Autodesk Fusion 360 part; units mm, degrees
(part 2 of 2)
  arc A538 (8.0741, 18.3325) -> (8.0737, 18.1922) centre (8.8652, 18.2601) ccw
  arc A539 (8.1154, 18.5393) -> (8.0741, 18.3325) centre (9.07, 18.2414) ccw
  arc A540 (8.1154, 18.5393) -> (8.0313, 18.7219) centre (7.9722, 18.584) ccw
  arc A541 (8.0313, 18.7219) -> (7.5594, 18.9174) centre (0, 0) ccw
  arc A542 (7.5594, 18.9174) -> (7.3708, 18.8477) centre (7.5037, 18.7781) ccw
  arc A543 (7.2538, 18.6723) -> (7.3708, 18.8477) centre (6.4851, 19.312) ccw
  arc A544 (7.1548, 18.5728) -> (7.2538, 18.6723) centre (6.6432, 19.1805) ccw
  arc A545 (6.6104, 18.4748) -> (7.1548, 18.5728) centre (6.7974, 18.9974) ccw
  arc A546 (6.2517, 18.896) -> (6.6104, 18.4748) centre (6.7974, 18.9974) ccw
  arc A547 (6.2384, 19.0357) -> (6.2517, 18.896) centre (7.0327, 19.0411) ccw
  arc A548 (6.2592, 19.2455) -> (6.2384, 19.0357) centre (7.2383, 19.0425) ccw
  arc A549 (6.2592, 19.2455) -> (6.1576, 19.419) centre (6.1123, 19.276) ccw
  arc A550 (6.1576, 19.419) -> (5.6687, 19.5672) centre (0, 0) ccw
  arc A551 (5.6687, 19.5672) -> (5.4879, 19.4795) centre (5.627, 19.4232) ccw
  arc A552 (5.3886, 19.2934) -> (5.4879, 19.4795) centre (4.561, 19.8547) ccw
  arc A553 (5.2999, 19.1847) -> (5.3886, 19.2934) centre (4.7312, 19.7393) ccw
  arc A554 (4.7677, 19.0338) -> (5.2999, 19.1847) centre (4.9026, 19.5722) ccw
  arc A555 (4.3695, 19.4177) -> (4.7677, 19.0338) centre (4.9026, 19.5722) ccw
  arc A556 (4.3425, 19.5555) -> (4.3695, 19.4177) centre (5.1325, 19.6388) ccw
  arc A557 (4.3426, 19.7663) -> (4.3425, 19.5555) centre (5.337, 19.6603) ccw
  arc A558 (4.3426, 19.7663) -> (4.2245, 19.929) centre (4.1935, 19.7822) ccw
  arc A559 (4.2245, 19.929) -> (3.7235, 20.0287) centre (0, 0) ccw
  arc A560 (3.7235, 20.0287) -> (3.5522, 19.9236) centre (3.6961, 19.8812) ccw
  arc A561 (3.4716, 19.7287) -> (3.5522, 19.9236) centre (2.5929, 20.2061) ccw
  arc A562 (3.394, 19.6118) -> (3.4716, 19.7287) centre (2.7736, 20.108) ccw
  arc A563 (2.8791, 19.4095) -> (3.394, 19.6118) centre (2.9606, 19.9584) ccw
  arc A564 (2.4452, 19.7525) -> (2.8791, 19.4095) centre (2.9606, 19.9584) ccw
  arc A565 (2.4048, 19.887) -> (2.4452, 19.7525) centre (3.1828, 20.0473) ccw
  arc A566 (2.3843, 20.0968) -> (2.4048, 19.887) centre (3.3842, 20.0888) ccw
  arc A567 (2.3843, 20.0968) -> (2.2508, 20.2471) centre (2.2343, 20.098) ccw
  arc A568 (2.2508, 20.2471) -> (1.7424, 20.2972) centre (0, 0) ccw
  arc A569 (1.7424, 20.2972) -> (1.5822, 20.1758) centre (1.7296, 20.1477) ccw
  arc A570 (1.5211, 19.974) -> (1.5822, 20.1758) centre (0.5999, 20.363) ccw
  arc A571 (1.4553, 19.85) -> (1.5211, 19.974) centre (0.7893, 20.283) ccw
  arc A572 (0.9628, 19.5982) -> (1.4553, 19.85) centre (0.99, 20.1525) ccw
  arc A573 (0.4973, 19.8971) -> (0.9628, 19.5982) centre (0.99, 20.1525) ccw
  arc A574 (0.444, 20.0269) -> (0.4973, 19.8971) centre (1.2025, 20.2627) ccw
  arc A575 (0.403, 20.2337) -> (0.444, 20.0269) centre (1.3989, 20.3237) ccw
  circle A576 centre (0, 0) radius 21.5
  dimension "d56" = 43
  constraint concentric A1 A576
  measures "d56" diameter of A576
extrude "Extruir10" add sketch "Boceto8" along normal blind 2 contours A0 A1 A2 A3 A4 A5 A6 A7 A8 A9 A10 A11 A12 A13 A14 A15 A16 A17 A18 A19 A20 A21 A22 A23 A24 A25 A26 A27 A28 A29 A30 A31 A32 A33 A34 A35 A36 A37 A38 A39 A40 A41 A42 A43 A44 A45 A46 A47 A48 A49 A50 A51 A52 A53 A54 A55 A56 A57 A58 A59 A60 A61 A62 A63 A64 A65 A66 A67 A68 A69 A70 A71 A72 A73 A74 A75 A76 A77 A78 A79 A80 A81 A82 A83 A84 A85 A86 A87 A88 A89 A90 A91 A92 A93 A94 A95 A96 A97 A98 A99 A100 A101 A102 A103 A104 A105 A106 A107 A108 A109 A110 A111 A112 A113 A114 A115 A116 A117 A118 A119 A120 A121 A122 A123 A124 A125 A126 A127 A128 A129 A130 A131 A132 A133 A134 A135 A136 A137 A138 A139 A140 A141 A142 A143 A144 A145 A146 A147 A148 A149 A150 A151 A152 A153 A154 A155 A156 A157 A158 A159 A160 A161 A162 A163 A164 A165 A166 A167 A168 A169 A170 A171 A172 A173 A174 A175 A176 A177 A178 A179 A180 A181 A182 A183 A184 A185 A186 A187 A188 A189 A190 A191 A192 A193 A194 A195 A196 A197 A198 A199 A200 A201 A202 A203 A204 A205 A206 A207 A208 A209 A210 A211 A212 A213 A214 A215 A216 A217 A218 A219 A220 A221 A222 A223 A224 A225 A226 A227 A228 A229 A230 A231 A232 A233 A234 A235 A236 A237 A238 A239 A240 A241 A242 A243 A244 A245 A246 A247 A248 A249 A250 A251 A252 A253 A254 A255 A256 A257 A258 A259 A260 A261 A262 A263 A264 A265 A266 A267 A268 A269 A270 A271 A272 A273 A274 A275 A276 A277 A278 A279 A280 A281 A282 A283 A284 A285 A286 A287 A288 A289 A290 A291 A292 A293 A294 A295 A296 A297 A298 A299 A300 A301 A302 A303 A304 A305 A306 A307 A308 A309 A310 A311 A312 A313 A314 A315 A316 A317 A318 A319 A320 A321 A322 A323 A324 A325 A326 A327 A328 A329 A330 A331 A332 A333 A334 A335 A336 A337 A338 A339 A340 A341 A342 A343 A344 A345 A346 A347 A348 A349 A350 A351 A352 A353 A354 A355 A356 A357 A358 A359 A360 A361 A362 A363 A364 A365 A366 A367 A368 A369 A370 A371 A372 A373 A374 A375 A376 A377 A378 A379 A380 A381 A382 A383 A384 A385 A386 A387 A388 A389 A390 A391 A392 A393 A394 A395 A396 A397 A398 A399 A400 A401 A402 A403 A404 A405 A406 A407 A408 A409 A410 A411 A412 A413 A414 A415 A416 A417 A418 A419 A420 A421 A422 A423 A424 A425 A426 A427 A428 A429 A430 A431 A432 A433 A434 A435 A436 A437 A438 A439 A440 A441 A442 A443 A444 A445 A446 A447 A448 A449 A450 A451 A452 A453 A454 A455 A456 A457 A458 A459 A460 A461 A462 A463 A464 A465 A466 A467 A468 A469 A470 A471 A472 A473 A474 A475 A476 A477 A478 A479 A480 A481 A482 A483 A484 A485 A486 A487 A488 A489 A490 A491 A492 A493 A494 A495 A496 A497 A498 A499 A500 A501 A502 A503 A504 A505 A506 A507 A508 A509 A510 A511 A512 A513 A514 A515 A516 A517 A518 A519 A520 A521 A522 A523 A524 A525 A526 A527 A528 A529 A530 A531 A532 A533 A534 A535 A536 A537 A538 A539 A540 A541 A542 A543 A544 A545 A546 A547 A548 A549 A550 A551 A552 A553 A554 A555 A556 A557 A558 A559 A560 A561 A562 A563 A564 A565 A566 A567 A568 A569 A570 A571 A572 A573 A574 A575 | A576 bodies 1
sketch "Boceto9" plane through (0, 0, 0) normal (0, 0, 1) x (1, 0, 0)
  circle A0 centre (0, 0) radius 21.5
  dimension "d59" = 43
  constraint coincident A0.centre origin
  measures "d59" diameter of A0
extrude "Extruir11" add sketch "Boceto9" against normal blind 7 bodies 1
move_body "Desplazar1" bodies 1 to x (1, 0, 0) y (0, 1, 0) z (0, 0, 1) at (0, 0, 7)
ref_plane "PlanoDeObra1" through (0, -21.5, 3.4245) normal (0, -1, 0) x (1, 0, 0)
sketch "Boceto10" plane through (0, -21.5, 3.4245) normal (0, -1, 0) x (1, 0, 0)
sketch "Boceto11" plane through (0, 0, 0) normal (0, 0, 1) x (1, 0, 0)
  circle A0 centre (0, 0) radius 15
  dimension "d63" = 30
  constraint coincident A0.centre origin
  measures "d63" diameter of A0
extrude "Extruir12" cut sketch "Boceto11" along normal blind 14 bodies 1
extrude "Extruir13" cut 1 faces at (3.8315, 5.6199, 14) along direction (0, 0, 1) blind 6 on bodies 1 bodies 1
extrude "Extruir14" add 1 faces at (-19.2533, 1.0681, 20) along direction (0, 0, 1) blind 9 on bodies 1 bodies 1
extrude "Extruir15" add 1 faces at (19.2533, -1.0681, 0) along direction (0, 0, -1) blind 3 on bodies 1 bodies 1
extrude "Extruir16" cut 1 faces at (-19.2533, 1.0681, 29) along direction (0, 0, -1) blind 1 on bodies 1 bodies 1
ref_plane "PlanoDeObra2" through (0, -21.5, 23.977) normal (0, -1, 0) x (-1, 0, 0)
sketch "Boceto12" plane through (0, -21.5, 23.977) normal (0, -1, 0) x (1, 0, 0)
  line L0 (2, -1) -> (0, -1)
  line L1 (0, -1) -> (0, 4)
  constraint horizontal L0
  constraint vertical L1
hole "Agujero2" at (0, -21.5, 22.977) direction (0, 1, 0) diameter 2.529 depth 9 tip angle 118 bodies 1
thread "Rosca2" "ISO Metric profile 3.0 M3x0.5 6H"
ref_plane "PlanoDeObra3" through (0, 21.5, 3.3729) normal (0, 1, 0) x (-1, 0, 0)
sketch "Boceto13" plane through (0, 21.5, 3.3729) normal (0, 1, 0) x (1, 0, 0)
move_body "Desplazar2" bodies 1 to x (1, 0, 0) y (0, 1, 0) z (0, 0, 1) at (0, 0, 3)
ref_plane "PlanoDeObra4" through (0, 21.5, 3.6034) normal (0, 1, 0) x (-1, 0, 0)
sketch "Boceto14" plane through (0, 21.5, 3.6034) normal (0, 1, 0) x (1, 0, 0)
sketch "Boceto15" plane through (0, 0, 0) normal (0, 1, 0) x (1, 0, 0)
  line L0 (0, 0) -> (-2, 0)
  line L1 (-2, 0) -> (-2, -5)
  line L2 (-2, -5) -> (0, -5)
  constraint horizontal L0
  constraint vertical L1
  constraint horizontal L2
  constraint coincident L0.start origin
ref_plane "PlanoDeObra5" through (0, 21.5, 4.5201) normal (0, 1, 0) x (-1, 0, 0)
sketch "Boceto16" plane through (0, 21.5, 4.5201) normal (0, 1, 0) x (1, 0, 0)
move_body "Desplazar3" bodies 1 to x (1, 0, 0) y (0, 1, 0) z (0, 0, 1) at (0, -21.5, 0)
hole "Agujero3" at (0, 0, 5) direction (0, -1, 0) diameter 2.529 depth 9 tip angle 118 bodies 1
thread "Rosca3" "ISO Metric profile 3.0 M3x0.5 6H"
copy_body "Cuerpo - > Comp.3" bodies 1 removing the originals makes body 65 in component "Component"
component "Component" placed x (1, 0, 0) y (0, 1, 0) z (0, 0, 1) at (0, 0, 0)
equation "NumTeeth = 64"
equation "ToothPitch = 2 mm"
equation "PullyDi = ToothPitch * NumTeeth / PI"
equation "ToothAng = ( 360 / NumTeeth ) * 1 deg"
equation "TransOffsetAngle = ToothAng * 0.2"
equation "Shoulder_Radius = 0.15 mm"
equation "Root_Radius = 0.555 mm"
equation "Trans_Radius = 1 mm"
equation "ToothHeight = 0.75 mm"
equation "PLD = 0.254 mm"
equation "d21 = ToothAng / 2"
equation "d22 = TransOffsetAngle"
equation "d23 = ToothHeight"
equation "d24 = PullyDi"
equation "d25 = Root_Radius"
equation "d26 = Trans_Radius * 2"
equation "d27 = 2 * Shoulder_Radius"
equation "d31 = ToothHeight"
